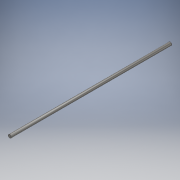
# Autodesk Inventor part: 8x400 Linear Guide
Saved by Autodesk Inventor 2019 (Build 230136000, 136)
## iProperties
Created: 2018-06-16
Part Number: 8x400 Linear Guide
Material: Stainless Steel
Document SubType Name: Modeling
Designer: Richard
Density: 8 g/cm^3
Appearance: Semi-Polished
Author: Richard
Autodesk Inventor part; units mm, degrees
ref_plane "YZ Plane" through (0, 0, 0) normal (1, 0, 0) x (0, 1, 0)
ref_plane "XZ Plane" through (0, 0, 0) normal (0, 1, 0) x (-1, 0, 0)
ref_plane "XY Plane" through (0, 0, 0) normal (0, 0, 1) x (1, 0, 0)
sketch "Sketch1" plane through (0, 0, 0) normal (0, 0, 1) x (1, 0, 0)
  circle A0 centre (0, 0) radius 4
  dimension "d0" = 8
  constraints: 1 centre point, 1 coincident
  measures "d0" diameter of A0
extrude "Extrusion1" add sketch "Sketch1" along normal mid plane 400
chamfer "Chamfer1" distance 0.635 angle 45 2 edges at (-4, 0, 200) (-4, 0, -200)
body "Solid1"
